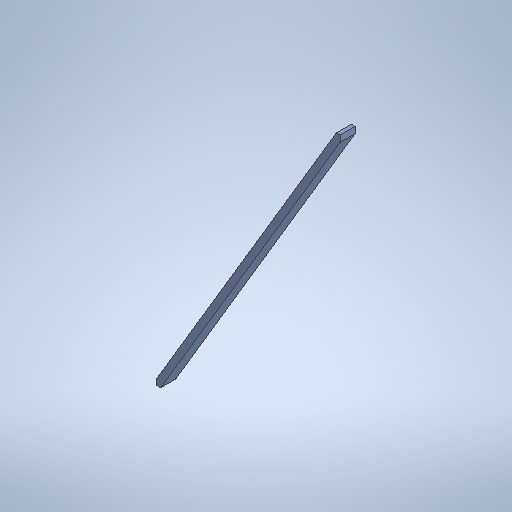
# Autodesk Inventor part: Part11
Saved by Autodesk Inventor 2025.1 (Build 291241020, 241B)
## iProperties
Created: 2024-09-16
Part Number: Part11
Material: Generic
Document SubType Name: Modeling
Designer: User
Density: 1 g/cm^3
Appearance: Default
Author: User
Autodesk Inventor part; units mm, degrees
ref_plane "YZ Plane" through (0, 0, 0) normal (1, 0, 0) x (0, 1, 0)
ref_plane "XZ Plane" through (0, 0, 0) normal (0, 1, 0) x (-1, 0, 0)
ref_plane "XY Plane" through (0, 0, 0) normal (0, 0, 1) x (1, 0, 0)
ref_plane "Work Plane1" through (0, 0, 0) normal (0, 0, 1) x (1, 0, 0)
sketch "Sketch1" plane through (0, 0, 0) normal (0, 0, 1) x (1, 0, 0)
  line L0 (-1241.3549, -38.1) -> (-1219.2, -38.1)
  line L1 (-1219.2, -38.1) -> (-1219.2, -75.4135)
  line L2 (-1219.2, -75.4135) -> (-2282.8951, -1866.9)
  line L3 (-2282.8951, -1866.9) -> (-2305.05, -1866.9)
  line L4 (-2305.05, -1866.9) -> (-2305.05, -1829.5865)
  line L5 (-2305.05, -1829.5865) -> (-1241.3549, -38.1)
  point P0 (0, 0)
  constraints: 12 end point, 2 parallel, 2 perpendicular, 1 horizontal, 6 other
extrude "Extrusion1" add sketch "Sketch1" against normal blind 88.9
body "Solid1"
